squeegee_hanger (Autodesk Fusion 360 design; units mm, degrees)
Autodesk Fusion 360 part; units mm, degrees
sketch "Sketch1" plane through (0, 0, 0) normal (0, 1, 0) x (1, 0, 0)
  line L0 (-30, -20) -> (30, -20)
  arc A0 (30, -20) -> (30, 20) centre (30, 0) ccw
  line L1 (30, 20) -> (-30, 20)
  arc A1 (-30, 20) -> (-30, -20) centre (-30, 0) ccw
  line L2 (-30, 0) -> (30, 0) construction
  circle A2 centre (-30, 0) radius 8
  circle A3 centre (30, 0) radius 8
  dimension "d1" = 40
  dimension "d2" = 60
  dimension "d3" = 16
  dimension "d4" = 16
  constraint tangent L0 A0
  constraint tangent A0 L1
  constraint parallel L0 L1
  constraint tangent L1 A1
  constraint tangent L0 A1
  constraint horizontal L2
  constraint midpoint origin L2
  constraint concentric A1 A2
  constraint concentric A0 A3
  measures "d1" distance of L0 L1
  measures "d2" distance of L0.start L0.end
  measures "d3" diameter of A3
  measures "d4" diameter of A2
extrude "Extrude1" add sketch "Sketch1" along normal blind 5 contours L0 A0 L1 A1 | A2 | A3
ref_plane "WorkPlane1" through (30, 0, 0) normal (1, 0, 0) x (0, 1, 0)
sketch "Sketch2" plane through (30, 0, 0) normal (1, 0, 0) x (0, 1, 0)
  spline S0 degree 5 poles (0, 0) (-0.9347, -0.0687) (-2.7839, -0.1732) (-5.497, -0.2316) (-8.9914, -0.1094) (-13.1398, 0.3999) (-17.048, 1.2992) (-20.695, 2.6229) (-24.0664, 4.3941) (-27.1693, 6.6013) (-30.0225, 9.2141) (-32.121, 11.6034) (-33.5976, 13.5531) (-34.5396, 14.9219) (-35, 15.6235) knots 0 0 0 0 0 0 0.1 0.2 0.3 0.4 0.5 0.6 0.7 0.8 0.9 1 1 1 1 1 1
  point P0 (-21.1718, 2.982)
  dimension "d14" = 35
  constraint coincident S0.start origin
  measures "d14" distance of S0.end S0.start
sweep "Sweep1" add profiles "Sketch1" path "Sketch2" along S0 section 1 contours A2 | A3
fillet "Fillet1" radius 5 2 edges at (-37.4586, -37.5285, 14.218) (22.5414, -37.5285, 14.218)
equation "d4 = d3"
